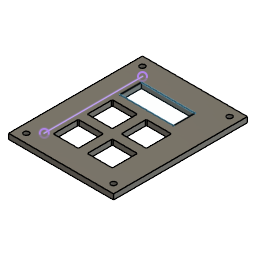
lid (Autodesk Fusion 360 design; units mm, degrees)
part number: 2026-03-17-22-19-55-551
Autodesk Fusion 360 part; units mm, degrees
sketch "Sketch1" plane through (0, 0, 0) normal (0, 1, 0) x (1, 0, 0)
  line L0 (0, 0) -> (58.8, 0)
  line L1 (58.8, 0) -> (58.8, 75)
  line L2 (58.8, 75) -> (0, 75)
  line L3 (0, 75) -> (0, 0)
  dimension "d1" = 58.8
  dimension "d2" = 75
  constraint horizontal L0
  constraint vertical L1
  constraint horizontal L2
  constraint vertical L3
  constraint coincident L0.start L3.end
  measures "d1" distance of L1.end L2.end
  measures "d2" distance of L0.end L1.end
extrude "Extrude1" add sketch "Sketch1" along normal blind 3
sketch "Sketch2" plane through (0, 3, 0) normal (0, 1, 0) x (-1, 0, 0)
  line L0 (0, -75) -> (0, 0)
  line L1 (0, 0) -> (-58.8, 0)
  line L2 (-58.8, 0) -> (-58.8, -75)
  line L3 (-58.8, -75) -> (0, -75)
  line L4 (-10, -65) -> (-48.8, -65)
  line L5 (-48.8, -65) -> (-48.8, -10)
  line L6 (-48.8, -10) -> (-10, -10)
  line L7 (-10, -10) -> (-10, -65)
  dimension "d5" = 10
  dimension "d6" = 10
  dimension "d7" = 10
  dimension "d8" = 10
  constraint horizontal L4
  constraint vertical L5
  constraint horizontal L6
  constraint vertical L7
  measures "d5" distance of L1 L6
  measures "d6" distance of L3 L4
  measures "d7" distance of L2 L5
  measures "d8" distance of L0 L7
sketch "plate-2026-03-17T21_53_59.045Z" plane through (0, 3, 0) normal (0, 1, 0) x (0, 0, 1)
  line L0 (-44.8182, 45.8566) -> (-31.8182, 45.8566)
  line L1 (-44.8182, 31.8566) -> (-31.8182, 31.8566)
  line L2 (-45.3182, 45.3566) -> (-45.3182, 32.3566)
  line L3 (-31.3182, 45.3566) -> (-31.3182, 32.3566)
  arc A0 (-44.8182, 45.8566) -> (-45.3182, 45.3566) centre (-44.8182, 45.3566) ccw
  arc A1 (-31.3182, 45.3566) -> (-31.8182, 45.8566) centre (-31.8182, 45.3566) ccw
  arc A2 (-45.3182, 32.3566) -> (-44.8182, 31.8566) centre (-44.8182, 32.3566) ccw
  arc A3 (-31.8182, 31.8566) -> (-31.3182, 32.3566) centre (-31.8182, 32.3566) ccw
  line L4 (-25.7682, 45.8566) -> (-12.7682, 45.8566)
  line L5 (-25.7682, 31.8566) -> (-12.7682, 31.8566)
  line L6 (-26.2682, 45.3566) -> (-26.2682, 32.3566)
  line L7 (-12.2682, 45.3566) -> (-12.2682, 32.3566)
  arc A4 (-25.7682, 45.8566) -> (-26.2682, 45.3566) centre (-25.7682, 45.3566) ccw
  arc A5 (-12.2682, 45.3566) -> (-12.7682, 45.8566) centre (-12.7682, 45.3566) ccw
  arc A6 (-26.2682, 32.3566) -> (-25.7682, 31.8566) centre (-25.7682, 32.3566) ccw
  arc A7 (-12.7682, 31.8566) -> (-12.2682, 32.3566) centre (-12.7682, 32.3566) ccw
  line L8 (-44.8182, 26.8066) -> (-31.8182, 26.8066)
  line L9 (-44.8182, 12.8066) -> (-31.8182, 12.8066)
  line L10 (-45.3182, 26.3066) -> (-45.3182, 13.3066)
  line L11 (-31.3182, 26.3066) -> (-31.3182, 13.3066)
  arc A8 (-44.8182, 26.8066) -> (-45.3182, 26.3066) centre (-44.8182, 26.3066) ccw
  arc A9 (-31.3182, 26.3066) -> (-31.8182, 26.8066) centre (-31.8182, 26.3066) ccw
  arc A10 (-45.3182, 13.3066) -> (-44.8182, 12.8066) centre (-44.8182, 13.3066) ccw
  arc A11 (-31.8182, 12.8066) -> (-31.3182, 13.3066) centre (-31.8182, 13.3066) ccw
  line L12 (-25.7682, 26.8066) -> (-12.7682, 26.8066)
  line L13 (-25.7682, 12.8066) -> (-12.7682, 12.8066)
  line L14 (-26.2682, 26.3066) -> (-26.2682, 13.3066)
  line L15 (-12.2682, 26.3066) -> (-12.2682, 13.3066)
  arc A12 (-25.7682, 26.8066) -> (-26.2682, 26.3066) centre (-25.7682, 26.3066) ccw
  arc A13 (-12.2682, 26.3066) -> (-12.7682, 26.8066) centre (-12.7682, 26.3066) ccw
  arc A14 (-26.2682, 13.3066) -> (-25.7682, 12.8066) centre (-25.7682, 13.3066) ccw
  arc A15 (-12.7682, 12.8066) -> (-12.2682, 13.3066) centre (-12.7682, 13.3066) ccw
  line L16 (-47.8432, 10.2816) -> (-9.7432, 10.2816)
  line L17 (-47.8432, 48.3816) -> (-9.7432, 48.3816)
  line L18 (-47.8432, 10.2816) -> (-47.8432, 48.3816)
  line L19 (-9.7432, 10.2816) -> (-9.7432, 48.3816)
extrude "Extrude2" cut sketch "plate-2026-03-17T21_53_59.045Z" against normal blind 3 contours L0 L1 L2 L3 A0 A1 A2 A3 | L4 L5 L6 L7 A4 A5 A6 A7 | L8 L9 L10 L11 A8 A9 A10 A11 | L12 L13 L14 L15 A12 A13 A14 A15
sketch "Sketch4" plane through (0, 3, 0) normal (0, 1, 0) x (-1, 0, 0)
  line L0 (-12.5, -61.899) -> (-42.5, -61.899)
  line L1 (-42.5, -61.899) -> (-42.5, -49.899)
  line L2 (-42.5, -49.899) -> (-12.5, -49.899)
  line L3 (-12.5, -49.899) -> (-12.5, -61.899)
  line L4 (-10, -10) -> (-10, -65)
  dimension "d11" = 12
  dimension "d12" = 30
  dimension "d13" = 2.5
  constraint horizontal L0
  constraint vertical L1
  constraint horizontal L2
  constraint vertical L3
  measures "d11" distance of L0.start L2.end
  measures "d12" distance of L0.start L0.end
  measures "d13" distance of L3 L4
extrude "Extrude3" cut sketch "Sketch4" against normal blind 3
sketch "Sketch5" plane through (0, 3, 0) normal (0, 1, 0) x (-1, 0, 0)
  circle A0 centre (-5, -70) radius 1.45
  circle A1 centre (-5, -5) radius 1.45
  circle A2 centre (-53.8, -70) radius 1.45
  circle A3 centre (-53.8, -5) radius 1.45
  line L0 (-58.8, -75) -> (0, -75)
  line L1 (0, -75) -> (0, 0)
  line L2 (0, 0) -> (-58.8, 0)
  line L3 (-58.8, 0) -> (-58.8, -75)
  dimension "d16" = 2.9
  dimension "d17" = 2.9
  dimension "d18" = 2.9
  dimension "d19" = 2.9
  dimension "d20" = 5
  dimension "d21" = 5
  dimension "d22" = 5
  dimension "d23" = 5
  dimension "d24" = 5
  dimension "d25" = 5
  dimension "d26" = 5
  dimension "d27" = 5
  measures "d16" diameter of A0
  measures "d17" diameter of A1
  measures "d18" diameter of A2
  measures "d19" diameter of A3
  measures "d20" distance of A0.centre L0
  measures "d21" distance of A0.centre L1
  measures "d22" distance of A1.centre L2
  measures "d23" distance of A1.centre L1
  measures "d24" distance of A3.centre L2
  measures "d25" distance of A3.centre L3
  measures "d26" distance of A2.centre L3
  measures "d27" distance of A2.centre L0
extrude "Extrude4" cut sketch "Sketch5" against normal blind 3 contours A0 | A1 | A2 | A3
